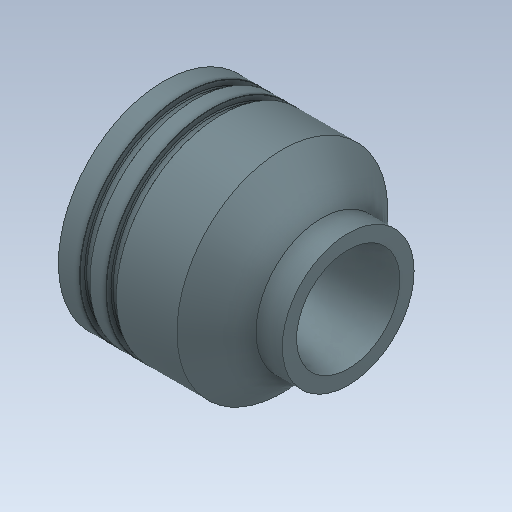
# Autodesk Inventor part: ODSY-0003-102
Saved by Autodesk Inventor 2021 (Build 250183000, 183)
## iProperties
Company: ERPL
Created: 2021-10-20
Material: Generic
Document SubType Name: Modeling
Designer: ALEX CLAY
Density: 2.26947 g/cm^3
Appearance: Lead
Mass: 1043.26 g
Surface Area: 482.002 cm^2
Volume: 459.694 cm^3
Project: ODYSSEY
Description: NOZZLE INSERT
Part Number: ODSY-0003-102
Author: ALEX CLAY
Revision Number: 00
Autodesk Inventor part; units mm, degrees
ref_plane "YZ Plane" through (0, 0, 0) normal (1, 0, 0) x (0, 1, 0)
ref_plane "XZ Plane" through (0, 0, 0) normal (0, 1, 0) x (-1, 0, 0)
ref_plane "XY Plane" through (0, 0, 0) normal (0, 0, 1) x (1, 0, 0)
derived "Rao Nozzle.ipt"
sketch "Sketch1" plane through (0, 0, 0) normal (0, 0, 1) x (1, 0, 0)
  arc A0 (-9.5322, 13.2328) -> (0, 9.652) centre (0, 24.13) ccw
  arc A1 (0, 9.652) -> (1.3812, 9.9205) centre (0, 13.3391) ccw
  line L0 (-7.4701, 9.652) -> (9.7854, 9.652) construction
  line L1 (-9.5322, 13.2328) -> (-43.4241, 42.8795)
  arc A2 (41.2951, 21.3656) -> (1.3812, 9.9205) centre (75.7848, -174.2348) ccw
  line L2 (1.3812, 9.9205) -> (21.8378, 18.1855) construction
  line L3 (41.2951, 21.3656) -> (80.2352, 28.2318) construction
  line L4 (41.2951, 21.3656) -> (95.911, 21.3656) construction
  line L5 (-47.6049, 50.8) -> (41.2951, 50.8)
  line L6 (41.2951, 50.8) -> (41.2951, 21.3656)
  line L7 (-72.1769, 0) -> (123.9257, 0)
  arc A3 (-43.4241, 42.8795) -> (-47.6049, 44.45) centre (-47.6049, 38.1) ccw
  line L8 (-47.6049, 44.45) -> (-47.6049, 50.8)
  line L9 (41.2951, 31.75) -> (28.5951, 31.75)
  line L10 (28.5951, 31.75) -> (9.5451, 50.8)
  point P0 (0, 0)
revolve "Revolution1" add sketch "Sketch1" angle 360 about axis through (-10, 0, 0) along (1, 0, 0) contours L1 A3 L8 L5 L10 L9 L6 A2 A1 A0
sketch "Sketch2" plane through (0, 0, 0) normal (0, 1, 0) x (-1, 0, 0)
  line L0 (37.2798, -50.8) -> (32.53, -50.8)
  line L1 (32.53, -50.8) -> (32.53, -47.9806)
  line L2 (32.53, -47.9806) -> (37.2798, -47.9806)
  line L3 (37.2798, -47.9806) -> (37.2798, -50.8)
  line L4 (24.5798, -47.9806) -> (19.83, -47.9806)
  line L5 (19.83, -47.9806) -> (19.83, -50.8)
  line L6 (19.83, -50.8) -> (24.5798, -50.8)
  line L7 (24.5798, -50.8) -> (24.5798, -47.9806)
  line L8 (34.9049, -50.8) -> (34.9049, -97.9888) construction
  line L9 (22.2049, -50.8) -> (22.2049, -101.7212) construction
  line L10 (47.6049, 50.8) -> (47.6049, -50.8) projected
  line L11 (44.4878, 0) -> (-7.4146, 0) projected
  point P0 (0, 0)
  dimension "d2" = 4.7498
  dimension "d3" = 4.7498
  dimension "d4" = 2.8194
  dimension "d5" = 12.7
  dimension "d6" = 12.7
  constraints: 20 end point, 4 parallel, 2 collinear, 2 horizontal, 2 midpoint, 2 perpendicular, 2 vertical, 1 point on line
  measures "d2" distance of L0.start L0.end
  measures "d3" distance of L5.end L6.end
  measures "d4" distance of L4.end L5.end
  measures "d5" distance between parallel lines of L9 L8
  measures "d6" distance between parallel lines of L8 L10
revolve "Revolution2" cut sketch "Sketch2" angle 360 about axis through (-10, 0, 0) along (1, 0, 0)
fillet "Fillet1" radius 0.508 4 edges at (-19.83, 0, 47.9806) (-32.53, 0, 47.9806) (-24.5798, 0, 47.9806) (-37.2798, 0, 47.9806)
fillet "Fillet2" radius 0.127 4 edges at (-37.2798, -50.8, 0) (-32.53, -50.8, 0) (-24.5798, -50.8, 0) (-19.83, -50.8, 0)
ref_plane "Work Plane1" through (-34.9049, 0, 0) normal (-1, 0, 0) x (0, 0, 1)
ref_plane "Work Plane2" through (-22.2049, 0, 0) normal (1, 0, 0) x (0, 0, -1)
body "Solid1"
